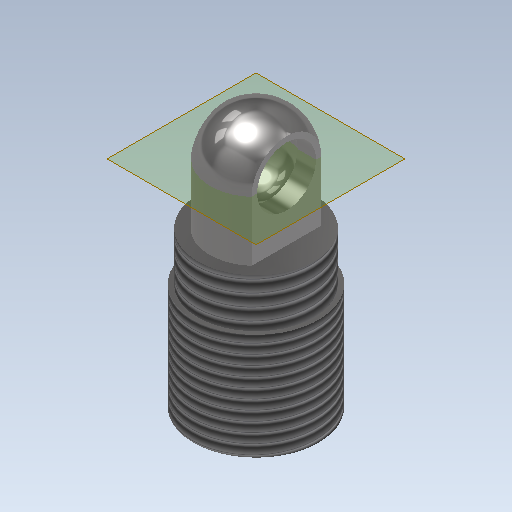
# Autodesk Inventor part: 500-106
Saved by Autodesk Inventor 2020 (Build 240168000, 168)
## iProperties
Created: 2015-04-18
Part Number: 500-106
Material: Stainless Steel
Document SubType Name: Modeling
Designer: Station9
Density: 8 g/cm^3
Appearance: Semi-Polished
Mass: 11.362 g
Surface Area: 15.6197 cm^2
Volume: 1.42024 cm^3
Author: Station9
Autodesk Inventor part; units mm, degrees
ref_plane "YZ Plane" through (0, 0, 0) normal (1, 0, 0) x (0, 1, 0)
ref_plane "XZ Plane" through (0, 0, 0) normal (0, 1, 0) x (-1, 0, 0)
ref_plane "XY Plane" through (0, 0, 0) normal (0, 0, 1) x (1, 0, 0)
sketch "Sketch1" plane through (0, 0, 0) normal (0, 1, 0) x (-1, 0, 0)
  circle A0 centre (0, 0) radius 6.4585
  dimension "d0" = 12.917
  constraints: 1 centre point, 1 coincident
  measures "d0" diameter of A0
extrude "Extrusion1" add sketch "Sketch1" along normal blind 11
sketch "Sketch2" plane through (0, 11, 0) normal (0, 1, 0) x (1, 0, 0)
  circle A0 centre (0, 0) radius 6.4585 projected
  circle A1 centre (0, 0) radius 6
  dimension "d3" = 12
  constraints: 1 centre point, 1 coincident
  measures "d3" diameter of A1
extrude "Extrusion2" add sketch "Sketch2" along normal blind 5 contours A1
sketch "Sketch3" plane through (0, 0, 0) normal (1, 0, 0) x (0, 1, 0)
  line L0 (16, -6) -> (16, 6) projected
  line L1 (16, -4.8) -> (22.2, -4.8)
  line L2 (22.2, 0) -> (16, 0)
  arc A0 (22.2, -4.8) -> (27, 0) centre (22.2, 0) ccw
  line L3 (0, 6.4585) -> (0, -6.4585) projected
  line L4 (22.2, 0) -> (27, 0)
  line L5 (16, 0) -> (27, 0)
  point P0 (0, 0)
  dimension "d7" = 4.8
  dimension "d13" = 22.2
  constraints: 8 end point, 2 horizontal, 2 point on circle, 2 point on line, 1 centre point, 1 collinear, 1 horizontal alignment, 1 midpoint, 1 tangent
  measures "d7" radius of A0
  measures "d13" distance from line of L3 L4.start
revolve "Revolution1" add sketch "Sketch3" angle 360 about axis through (0, 16, 0) along (0, 1, 0)
sketch "Sketch4" plane through (0, 16, 0) normal (0, 1, 0) x (1, 0, 0)
  circle A0 centre (0, 0) radius 4.8 projected
  circle A1 centre (0, 0) radius 6 projected
  line L0 (2.5, -11.2443) -> (-2.5, -11.2443)
  line L1 (-2.5, 11.2443) -> (2.5, 11.2443)
  line L2 (2.5, -11.2443) -> (-2.5, 11.2443) construction
  line L3 (-2.5, -11.2443) -> (2.5, 11.2443) construction
  circle A2 centre (0, 0) radius 4.8
  line L4 (2.5, 11.2443) -> (2.5, 5.4544)
  line L5 (3.1579, 3.6149) -> (3.1579, -3.6149)
  line L6 (-3.1579, -3.6149) -> (-3.1579, 3.6149)
  dimension "d9" = 5
  constraints: 14 end point, 4 point on circle, 3 parallel, 2 midpoint, 1 centre point, 1 coincident, 1 concentric, 1 horizontal, 1 perpendicular, 2 other
  measures "d9" distance of L1.start L1.end
extrude "Extrusion3" cut sketch "Sketch4" along normal blind 13.25 contours A0 L5 | L6 A0
hole "Hole1" at (3.1579, 22.2, 0) direction (-1, 0, 0) diameter 6.1 depth 8 tip angle 118
thread "Thread1" size "M14x1" class "6g" standard "ANSI Metric M Profile" full length
thread "Thread2" size "M12x1.25" class "6g" standard "ANSI Metric M Profile" full length
sketch "Sketch5" plane through (0, 0, 0) normal (0, -1, 0) x (1, 0, 0)
  circle A0 centre (0, 0) radius 6.4585 projected
  circle A1 centre (0, 0) radius 6
  dimension "d27" = 12
  constraints: 1 centre point, 1 coincident
  measures "d27" diameter of A1
hole "Hole2" at (0, 0, 0) direction (0, 1, 0) diameter 10.917 depth 10 thread size "M12x1" class "6H" standard "ISO Metric profile"
ref_plane "Work Plane1" through (-0.8421, 22.2, 0) normal (0, -1, 0) x (1, 0, 0)
sketch "Sketch6" plane through (-0.8421, 22.2, 0) normal (0, -1, 0) x (1, 0, 0)
  circle A0 centre (0.8421, 0) radius 3.3
  line L0 (4.1421, 0) -> (-2.4579, 0)
  line L1 (4, 3.05) -> (4, -3.05) projected
  line L2 (-8.1998, 0) -> (9.884, 0) projected
  dimension "d36" = 6.6
  constraints: 2 end point, 2 point on circle, 1 centre point, 1 coincident, 1 perpendicular
  measures "d36" diameter of A0
revolve "Revolution2" cut sketch "Sketch6" angle 360 about axis through (-0.8421, 22.2, 0) along (1, 0, 0) picked at (4.0262, 0.5339) picked at (-0.2745, 0.2585) contours L0 L1 A0 | L1 L0 A0
body "Solid1"
